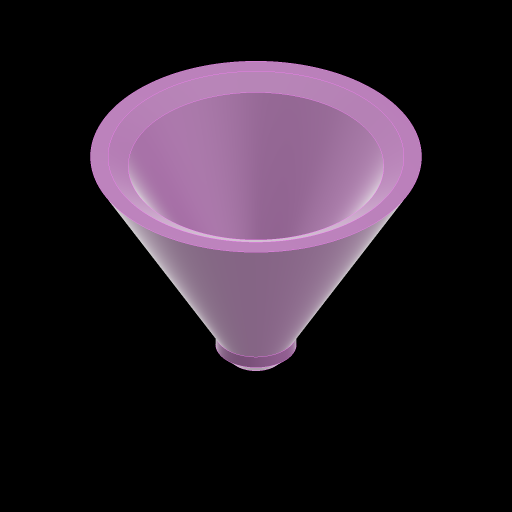
# Autodesk Inventor part: Funnel
Saved by Autodesk Inventor 2023 (Build 270158000, 158)
## iProperties
Created: 2023-09-12
Part Number: Funnel
Material: Generic
Document SubType Name: Modeling
Designer: tandu
Density: 1 g/cm^3
Appearance: Smooth - Purple
Author: tandu
Autodesk Inventor part; units mm, degrees
ref_plane "YZ Plane" through (0, 0, 0) normal (1, 0, 0) x (0, 1, 0)
ref_plane "XZ Plane" through (0, 0, 0) normal (0, 1, 0) x (-1, 0, 0)
ref_plane "XY Plane" through (0, 0, 0) normal (0, 0, 1) x (1, 0, 0)
sketch "Sketch1" plane through (0, 0, 0) normal (0, 0, 1) x (1, 0, 0)
  line L0 (1.27, 0) -> (1.27, 3.175)
  line L1 (1.27, 3.175) -> (12.7, 22.9723)
  line L2 (15.6329, 22.9723) -> (3.81, 2.4944)
  line L3 (3.81, 2.4944) -> (3.81, 0)
  line L4 (15.6329, 22.9723) -> (12.7, 22.9723)
  line L5 (3.81, 0) -> (1.27, 0)
  line L6 (0, -4.5945) -> (0, 27.5668) projected
  point P0 (0, 0)
  dimension "d0" = 2.54
  dimension "d1" = 1.27
  dimension "d2" = 3.175
  dimension "d3" = 12.7
  dimension "d4" = 150
  constraints: 12 end point, 3 horizontal alignment, 2 horizontal, 1 vertical, 1 other
  measures "d0" distance between parallel lines of L1 L2
  measures "d1" distance from line of point (0, 0) L0
  measures "d2" distance of L0.start L0.end
  measures "d3" horizontal distance of point (0, 0) L1.end
  measures "d4" angle of L0 L1
revolve "Revolution1" add sketch "Sketch1" angle 360 about axis through (0, -10, 0) along (0, 1, 0)
chamfer "Chamfer1" distance 1.27 angle 45 2 edges at (-12.7, 22.9723, 0) (-3.81, 0, 0)
body "Solid1"
